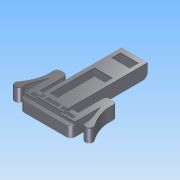
# Autodesk Inventor part: D2MG крепёж
Saved by Autodesk Inventor 2015 SP1 (Build 190203100, 203)
## iProperties
Created: 2017-11-06
Part Number: D2MG крепёж
Material: Типовые
Document SubType Name: Modeling
Designer: Влад
Density: 1 g/cm^3
Appearance: Гладкий — светло-серый
Author: Влад
Autodesk Inventor part; units mm, degrees
ref_plane "YZ Plane" through (0, 0, 0) normal (1, 0, 0) x (0, 1, 0)
ref_plane "XZ Plane" through (0, 0, 0) normal (0, 1, 0) x (-1, 0, 0)
ref_plane "XY Plane" through (0, 0, 0) normal (0, 0, 1) x (1, 0, 0)
sketch "Эскиз2" plane through (0, 0, 0) normal (0, 0, 1) x (1, 0, 0)
  line L0 (-14.25, 16.75) -> (14.25, -16.75) construction
  line L1 (14.25, 16.75) -> (-14.25, -16.75) construction
  line L2 (-14.6958, 16.5546) -> (14.3646, 16.5546) construction
  line L3 (14.3646, 16.5546) -> (14.3646, -16.928) construction
  line L4 (14.3646, -16.928) -> (-14.6958, -16.928) construction
  line L5 (-14.6958, -16.928) -> (-14.6958, 16.5546) construction
  line L6 (-0.2566, 16.1698) -> (4.6434, 16.1698)
  line L7 (4.6434, 16.1698) -> (4.6434, -11.7772)
  line L8 (4.6434, -11.7772) -> (6.7616, -11.7772)
  line L9 (6.7616, -11.7772) -> (6.7616, -2.8913)
  line L10 (8.2616, -1.3913) -> (9.334, -1.3913)
  line L11 (10.834, -2.8913) -> (10.834, -5.5103)
  line L12 (10.834, -5.5103) -> (11.4026, -9.4794) construction
  spline S0 degree 2 poles (10.834, -5.5103) (11.4026, -9.4794) (13.9221, -12.8762) knots 1 1 1 1.940289 1.940289 1.940289
  arc A0 (10.834, -2.8913) -> (9.334, -1.3913) centre (9.334, -2.8913) ccw
  arc A1 (8.2616, -1.3913) -> (6.7616, -2.8913) centre (8.2616, -2.8913) ccw
  circle A2 centre (12.7752, -13.7269) radius 1.428
  line L13 (9.1793, -6.3314) -> (11.4381, -11.9589) construction
  line L14 (11.4381, -11.9589) -> (11.4381, -13.2254) construction
  spline S1 degree 2 poles (9.1793, -6.3314) (11.4381, -11.9589) (11.4381, -13.2254) knots 1 1 1 2 2 2
  line L15 (9.1793, -6.3314) -> (9.1793, -15.228)
  line L16 (-0.2566, 21.2759) -> (-0.2566, -20.1625) construction
  line L17 (7.4793, -16.928) -> (-0.2566, -16.928)
  arc A3 (7.4793, -16.928) -> (9.1793, -15.228) centre (7.4793, -15.228) ccw
  line L18 (11.4026, -9.4794) -> (13.9221, -12.8762) construction
  line L19 (-0.2566, -14.7133) -> (2.2143, -14.7133)
  line L20 (2.2143, -14.7133) -> (2.2143, -13.3042)
  line L21 (2.2143, -13.3042) -> (-0.2566, -13.3042)
  line L22 (2.9887, -13.3042) -> (2.9887, -14.7133)
  line L23 (2.9887, -14.7133) -> (7.6349, -14.7133)
  line L24 (7.6349, -14.7133) -> (7.6349, -13.3042)
  line L25 (7.6349, -13.3042) -> (2.9887, -13.3042)
  line L26 (-0.2566, 4.5188) -> (3.0342, 4.5188)
  line L27 (3.0342, 4.5188) -> (3.0342, -11.7772)
  line L28 (3.0342, -11.7772) -> (2.2143, -11.7772)
  line L29 (2.2143, -11.7772) -> (2.2143, 3.7353)
  line L30 (2.2143, 3.7353) -> (-0.2566, 3.7353)
  line L31 (-0.2566, 3.4757) -> (1.8788, 3.4757)
  line L32 (1.8788, 3.4757) -> (1.8788, -11.7772)
  line L33 (1.8788, -11.7772) -> (-0.2566, -11.7772)
  line L34 (-0.2566, 14.0967) -> (3.0342, 14.0967)
  line L35 (3.0342, 14.0967) -> (3.0342, 10.9676)
  line L36 (3.0342, 10.9676) -> (-0.2566, 10.9676)
  line L37 (-0.2566, 16.1698) -> (-5.1566, 16.1698)
  line L38 (-5.1566, 16.1698) -> (-5.1566, -11.7772)
  line L39 (-5.1566, -11.7772) -> (-7.2749, -11.7772)
  line L40 (-7.2749, -11.7772) -> (-7.2749, -2.8913)
  line L41 (-8.7749, -1.3913) -> (-9.8473, -1.3913)
  line L42 (-11.3473, -2.8913) -> (-11.3473, -5.5103)
  line L43 (-11.3473, -5.5103) -> (-11.9159, -9.4794) construction
  spline S2 degree 2 poles (-11.3473, -5.5103) (-11.9159, -9.4794) (-14.4354, -12.8762) knots 1 1 1 1.940289 1.940289 1.940289
  arc A4 (-9.8473, -1.3913) -> (-11.3473, -2.8913) centre (-9.8473, -2.8913) ccw
  arc A5 (-7.2749, -2.8913) -> (-8.7749, -1.3913) centre (-8.7749, -2.8913) ccw
  circle A6 centre (-13.2885, -13.7269) radius 1.428
  line L44 (-9.6926, -6.3314) -> (-11.9514, -11.9589) construction
  line L45 (-11.9514, -11.9589) -> (-11.9514, -13.2254) construction
  spline S3 degree 2 poles (-9.6926, -6.3314) (-11.9514, -11.9589) (-11.9514, -13.2254) knots 1 1 1 2 2 2
  line L46 (-9.6926, -6.3314) -> (-9.6926, -15.228)
  line L47 (-7.9926, -16.928) -> (-0.2566, -16.928)
  arc A7 (-9.6926, -15.228) -> (-7.9926, -16.928) centre (-7.9926, -15.228) ccw
  line L48 (-11.9159, -9.4794) -> (-14.4354, -12.8762) construction
  line L49 (-0.2566, -14.7133) -> (-2.7276, -14.7133)
  line L50 (-2.7276, -14.7133) -> (-2.7276, -13.3042)
  line L51 (-2.7276, -13.3042) -> (-0.2566, -13.3042)
  line L52 (-3.502, -13.3042) -> (-3.502, -14.7133)
  line L53 (-3.502, -14.7133) -> (-8.1482, -14.7133)
  line L54 (-8.1482, -14.7133) -> (-8.1482, -13.3042)
  line L55 (-8.1482, -13.3042) -> (-3.502, -13.3042)
  line L56 (-0.2566, 4.5188) -> (-3.5475, 4.5188)
  line L57 (-3.5475, 4.5188) -> (-3.5475, -11.7772)
  line L58 (-3.5475, -11.7772) -> (-2.7276, -11.7772)
  line L59 (-2.7276, -11.7772) -> (-2.7276, 3.7353)
  line L60 (-2.7276, 3.7353) -> (-0.2566, 3.7353)
  line L61 (-0.2566, 3.4757) -> (-2.3921, 3.4757)
  line L62 (-2.3921, 3.4757) -> (-2.3921, -11.7772)
  line L63 (-2.3921, -11.7772) -> (-0.2566, -11.7772)
  line L64 (-0.2566, 14.0967) -> (-3.5475, 14.0967)
  line L65 (-3.5475, 14.0967) -> (-3.5475, 10.9676)
  line L66 (-3.5475, 10.9676) -> (-0.2566, 10.9676)
  point P0 (0, 0)
  point P1 (0, 0)
  point P2 (9.1793, -16.928)
  point P3 (-0.5133, 0)
  point P4 (-14.7633, -16.75)
  point P5 (-14.7633, 16.75)
  point P6 (-0.5133, 0)
  point P7 (-9.6926, -16.928)
  dimension "d3" = 28.5
  dimension "d4" = 33.5
  dimension "d35" = 1.5
  dimension "d99" = 4.9
  dimension "d101" = 1.7
  constraints: 108 end point, 38 horizontal alignment, 22 point on line, 16 point on circle, 12 perpendicular, 8 centre point, 8 horizontal, 6 tangent, 5 equal radius, 2 coincident, 2 parallel, 1 midpoint, 28 other
  measures "d3" distance of L0.end L1.end
  measures "d4" distance of L1.start L0.end
  measures "d35" radius of A0
  measures "d101" radius of A3
extrude "Выдавливание1" add sketch "Эскиз2" along normal blind 5 contours L6 L7 L8 L9 A1 L10 A0 L11 S0 A2 S1 L15 A3 L17 L47 A7 L46 S3 A6 S2 L42 A4 L41 A5 L40 L39 L38 L37 | A2 | A6 | L31 L32 L33 L63 L62 L61
fillet "Сопряжение2" radius 2 1 edges at (-0.2566, 16.1698, 0)
sketch "Эскиз3" plane through (0, 0, 0) normal (0, 0, -1) x (-1, 0, 0)
  line L0 (-6.7616, -2.8913) -> (-6.7616, -11.7772) projected
  arc A0 (-6.7616, -2.8913) -> (-8.2616, -1.3913) centre (-8.2616, -2.8913) ccw projected
  line L1 (-9.334, -1.3913) -> (-8.2616, -1.3913) projected
  arc A1 (-9.334, -1.3913) -> (-10.834, -2.8913) centre (-9.334, -2.8913) ccw projected
  line L2 (-10.834, -5.5103) -> (-10.834, -2.8913) projected
  spline S0 degree 2 poles (-13.9221, -12.8762) (-11.4026, -9.4794) (-10.834, -5.5103) knots 0 0 0 1 1 1 projected
  arc A2 (-13.9221, -12.8762) -> (-11.4381, -13.2254) centre (-12.7752, -13.7269) ccw projected
  spline S1 degree 2 poles (-9.1793, -6.3314) (-11.4381, -11.9589) (-11.4381, -13.2254) knots 0 0 0 1 1 1 projected
  line L3 (-9.1793, -15.228) -> (-9.1793, -6.3314) projected
  arc A3 (-9.1793, -15.228) -> (-7.4793, -16.928) centre (-7.4793, -15.228) ccw projected
  line L4 (7.9926, -16.928) -> (-7.4793, -16.928) projected
  arc A4 (7.9926, -16.928) -> (9.6926, -15.228) centre (7.9926, -15.228) ccw projected
  line L5 (9.6926, -6.3314) -> (9.6926, -15.228) projected
  spline S2 degree 2 poles (11.9514, -13.2254) (11.9514, -11.9589) (9.6926, -6.3314) knots 0 0 0 1 1 1 projected
  arc A5 (11.9514, -13.2254) -> (14.4354, -12.8762) centre (13.2885, -13.7269) ccw projected
  spline S3 degree 2 poles (11.3473, -5.5103) (11.9159, -9.4794) (14.4354, -12.8762) knots 0 0 0 1 1 1 projected
  line L6 (11.3473, -2.8913) -> (11.3473, -5.5103) projected
  arc A6 (11.3473, -2.8913) -> (9.8473, -1.3913) centre (9.8473, -2.8913) ccw projected
  line L7 (8.7749, -1.3913) -> (9.8473, -1.3913) projected
  line L8 (7.2749, -11.7772) -> (7.2749, -2.8913) projected
  arc A7 (8.7749, -1.3913) -> (7.2749, -2.8913) centre (8.7749, -2.8913) ccw projected
  line L9 (5.1566, -11.7772) -> (7.2749, -11.7772) projected
  line L10 (3.502, -13.3042) -> (8.1482, -13.3042) projected
  line L11 (3.502, -14.7133) -> (3.502, -13.3042) projected
  line L12 (8.1482, -14.7133) -> (3.502, -14.7133) projected
  line L13 (8.1482, -13.3042) -> (8.1482, -14.7133) projected
  line L14 (2.7276, -13.3042) -> (2.7276, -14.7133) projected
  line L15 (-2.2143, -13.3042) -> (2.7276, -13.3042) projected
  line L16 (2.7276, -14.7133) -> (-2.2143, -14.7133) projected
  line L17 (-2.2143, -14.7133) -> (-2.2143, -13.3042) projected
  line L18 (-2.9887, -13.3042) -> (-2.9887, -14.7133) projected
  line L19 (-2.9887, -14.7133) -> (-7.6349, -14.7133) projected
  line L20 (-7.6349, -13.3042) -> (-2.9887, -13.3042) projected
  line L21 (-7.6349, -14.7133) -> (-7.6349, -13.3042) projected
  line L22 (-6.7616, -11.7772) -> (7.2749, -11.7772)
  point P0 (0, 0)
  constraints: 2 end point, 1 perpendicular, 4 other
extrude "Выдавливание2" add sketch "Эскиз3" along normal blind 1
sketch "Эскиз4" plane through (0, 0, 5) normal (0, 0, 1) x (1, 0, 0)
  arc A0 (-14.4354, -12.8762) -> (-11.9514, -13.2254) centre (-13.2885, -13.7269) ccw projected
  spline S0 degree 2 poles (-11.3473, -5.5103) (-11.9159, -9.4794) (-14.4354, -12.8762) knots 0 0 0 1 1 1 projected
  spline S1 degree 2 poles (-11.9514, -13.2254) (-11.9514, -11.9589) (-9.6926, -6.3314) knots 0 0 0 1 1 1 projected
  line L0 (-9.6926, -6.3314) -> (-9.6926, -15.228) projected
  arc A1 (-9.8473, -1.3913) -> (-11.3473, -2.8913) centre (-9.8473, -2.8913) ccw projected
  line L1 (-11.3473, -2.8913) -> (-11.3473, -5.5103) projected
  line L2 (-8.7749, -1.3913) -> (-9.8473, -1.3913) projected
  arc A2 (-7.2749, -2.8913) -> (-8.7749, -1.3913) centre (-8.7749, -2.8913) ccw projected
  line L3 (-7.2749, -11.7772) -> (-7.2749, -2.8913) projected
  line L4 (-8.1482, -14.7133) -> (-8.1482, -13.3042) projected
  line L5 (-3.502, -14.7133) -> (-8.1482, -14.7133) projected
  line L6 (-8.1482, -13.3042) -> (-3.502, -13.3042) projected
  line L7 (-3.502, -13.3042) -> (-3.502, -14.7133) projected
  arc A3 (-9.6926, -15.228) -> (-7.9926, -16.928) centre (-7.9926, -15.228) ccw projected
  line L8 (-7.9926, -16.928) -> (7.4793, -16.928) projected
  line L9 (-2.7276, -14.7133) -> (-2.7276, -13.3042) projected
  line L10 (2.2143, -14.7133) -> (-2.7276, -14.7133) projected
  line L11 (-2.7276, -13.3042) -> (2.2143, -13.3042) projected
  line L12 (2.2143, -13.3042) -> (2.2143, -14.7133) projected
  line L13 (2.9887, -14.7133) -> (2.9887, -13.3042) projected
  line L14 (7.6349, -14.7133) -> (2.9887, -14.7133) projected
  line L15 (2.9887, -13.3042) -> (7.6349, -13.3042) projected
  line L16 (7.6349, -13.3042) -> (7.6349, -14.7133) projected
  arc A4 (7.4793, -16.928) -> (9.1793, -15.228) centre (7.4793, -15.228) ccw projected
  line L17 (9.1793, -15.228) -> (9.1793, -6.3314) projected
  spline S2 degree 2 poles (9.1793, -6.3314) (11.4381, -11.9589) (11.4381, -13.2254) knots 0 0 0 1 1 1 projected
  arc A5 (11.4381, -13.2254) -> (13.9221, -12.8762) centre (12.7752, -13.7269) ccw projected
  spline S3 degree 2 poles (13.9221, -12.8762) (11.4026, -9.4794) (10.834, -5.5103) knots 0 0 0 1 1 1 projected
  line L18 (10.834, -5.5103) -> (10.834, -2.8913) projected
  arc A6 (10.834, -2.8913) -> (9.334, -1.3913) centre (9.334, -2.8913) ccw projected
  line L19 (9.334, -1.3913) -> (8.2616, -1.3913) projected
  arc A7 (8.2616, -1.3913) -> (6.7616, -2.8913) centre (8.2616, -2.8913) ccw projected
  line L20 (6.7616, -2.8913) -> (6.7616, -11.7772) projected
  line L21 (-7.2749, -11.7772) -> (6.7616, -11.7772)
  line L22 (-5.1566, -11.7772) -> (-7.2749, -11.7772) projected
  point P0 (0, 0)
  constraints: 2 end point, 1 collinear, 4 other
extrude "Выдавливание3" cut sketch "Эскиз4" against normal blind 1
sketch "Эскиз6" plane through (0, 0, 5) normal (0, 0, 1) x (1, 0, 0)
  line L0 (-5.1566, -11.7772) -> (-5.1566, -13.3042)
  line L1 (-5.1566, -13.3042) -> (-3.502, -13.3042)
  line L2 (-3.502, -13.3042) -> (-3.502, -14.7133)
  line L3 (-3.502, -14.7133) -> (-3.502, -13.3042) projected
  line L4 (-3.502, -14.7133) -> (-5.1566, -14.7133)
  line L5 (-5.1566, -14.7133) -> (-5.1566, -15.4633)
  line L6 (-5.1566, -15.4633) -> (4.6434, -15.4633)
  line L7 (4.6434, -11.7772) -> (-5.1566, -11.7772)
  line L8 (4.6434, -14.7133) -> (2.9887, -14.7133)
  line L9 (2.9887, -14.7133) -> (2.9887, -13.3042)
  line L10 (2.9887, -13.3042) -> (4.6434, -13.3042)
  line L11 (7.6349, -13.3042) -> (2.9887, -13.3042) projected
  line L12 (4.6434, -11.7772) -> (4.6434, -13.3042)
  line L13 (4.6434, -14.7133) -> (4.6434, -15.4633)
  line L14 (-2.7276, -14.7133) -> (2.2143, -14.7133)
  line L15 (2.2143, -14.7133) -> (2.2143, -13.3042)
  line L16 (2.2143, -13.3042) -> (-2.7276, -13.3042)
  line L17 (-2.7276, -13.3042) -> (-2.7276, -14.7133)
  point P0 (0, 0)
  dimension "d137" = 0.75
  constraints: 32 end point, 6 perpendicular, 3 equal length, 3 point on line, 3 vertical, 2 horizontal
  measures "d137" distance of L4.end L5.end
extrude "Выдавливание4" add sketch "Эскиз6" against normal blind 1
sketch "Эскиз7" plane through (0, 0, 4) normal (0, 0, 1) x (1, 0, 0)
  line L0 (-9.6762, -15.4633) -> (9.163, -15.4633)
  line L1 (-2.7276, -14.7133) -> (2.2143, -14.7133) projected
  arc A0 (-9.6926, -15.228) -> (-7.9926, -16.928) centre (-7.9926, -15.228) ccw projected
  line L2 (7.4793, -16.928) -> (-7.9926, -16.928) projected
  arc A1 (7.4793, -16.928) -> (9.1793, -15.228) centre (7.4793, -15.228) ccw projected
  point P0 (0, 0)
  dimension "d140" = 0.75
  constraints: 2 end point, 2 point on circle, 1 horizontal
  measures "d140" distance between parallel lines of L1 L0
extrude "Выдавливание5" cut sketch "Эскиз7" against normal blind 1
sketch "Эскиз8" plane through (0, 0, 5) normal (0, 0, 1) x (1, 0, 0)
  line L0 (-7.2749, -11.7772) -> (6.7616, -11.7772) projected
  line L1 (2.2143, 3.7353) -> (-2.7276, 3.7353)
  line L2 (-2.7276, 3.7353) -> (-2.7276, -11.7772)
  line L3 (-2.7276, -11.7772) -> (2.2143, -11.7772)
  line L4 (2.2143, -11.7772) -> (2.2143, 3.7353)
  point P0 (0, 0)
  constraints: 8 end point, 2 parallel, 1 horizontal, 1 perpendicular, 1 point on line
extrude "Выдавливание6" cut sketch "Эскиз8" against normal blind 2
sketch "Эскиз9" plane through (-2.7276, -11.7772, 0) normal (-1, 0, 0) x (0, 0, 1)
  line L0 (-1, 11.5126) -> (-1, 8.5126)
  line L1 (-1, 8.5126) -> (0, 8.5126)
  line L2 (0, 8.5126) -> (0, 15.5126)
  line L3 (-1, 11.5126) -> (0, 15.5126)
  point P0 (0, 11.7772)
  constraints: 8 end point, 1 parallel
extrude "Выдавливание7" add sketch "Эскиз9" against normal blind 4.9419
fillet "Сопряжение3" radius 0.2 21 edges at (4.6434, 15.584, 0.5858) (4.6434, 16.1698, 3.5) (4.6434, 1.4328, 5) (4.6434, 1.1963, 0) (-5.1566, 15.584, 0.5858) (-5.1566, 16.1698, 3.5) (-5.1566, 1.4328, 5) (-5.1566, 1.1963, 0) (-3.5475, 12.5322, 0) (-0.2566, 14.0967, 0) (-0.2566, 10.9676, 0) (3.0342, 12.5322, 0) (-0.2566, 14.0967, 5) (3.0342, 12.5322, 5) (-0.2566, 10.9676, 5) (-3.5475, 12.5322, 5) (3.0342, -3.6292, 5) (-0.2566, 4.5188, 5) (-3.5475, -3.6292, 5) (-0.2566, -11.7772, 5) (-0.2566, 16.1698, 5)
fillet "Сопряжение4" radius 0.5 1 edges at (-0.2566, 3.7353, 0)
fillet "Сопряжение5" radius 2 1 edges at (-0.2566, -0.2647, -1)
fillet "Сопряжение6" radius 0.2 49 edges at (12.974, -15.141, -1) (11.8903, -9.3363, -1) (10.3947, -1.8306, -1) (8.7978, -1.3913, -1) (7.201, -1.8306, -1) (6.7616, -7.3343, -1) (10.834, -4.2008, -1) (10.8734, -10.8687, -1) (8.6814, -16.43, -1) (-0.2566, -16.928, -1) (-9.1947, -16.43, -1) (-9.6926, -10.7797, -1) (9.1793, -10.7797, -1) (-11.3867, -10.8687, -1) (-12.4036, -9.3363, -1) (-13.4873, -15.141, -1) (-10.908, -1.8306, -1) (-9.3111, -1.3913, -1) (-7.7143, -1.8306, -1) (-7.2749, -7.3343, -1) (-11.3473, -4.2008, -1) (-7.7143, -1.8306, 4) (-9.3111, -1.3913, 4) (-10.908, -1.8306, 4) (-11.3473, -4.2008, 4) (-7.2749, -7.3343, 4) (-13.4873, -15.141, 4) (-12.4036, -9.3363, 4) (-11.3867, -10.8687, 4) (-9.6885, -15.3459, 4) (-9.6926, -10.7797, 4) (-9.6762, -15.4633, 3.5) (-7.4164, -15.4633, 4) (-0.2566, -15.4633, 5) (4.6434, -15.4633, 4.5) (-5.1566, -15.4633, 4.5) (6.9032, -15.4633, 4) (9.1752, -15.3459, 4) (9.1793, -10.7797, 4) (10.8734, -10.8687, 4) (11.8903, -9.3363, 4) (12.974, -15.141, 4) (10.3947, -1.8306, 4) (8.7978, -1.3913, 4) (7.201, -1.8306, 4) (6.7616, -7.3343, 4) (10.834, -4.2008, 4) (-6.2158, -11.7772, 4) (5.7025, -11.7772, 4)
